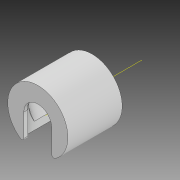
# Autodesk Inventor part: leur adapter2
Saved by Autodesk Inventor 2020 (Build 240168000, 168)
## iProperties
Created: 2020-08-02
Part Number: leur adapter2
Material: Generic
Document SubType Name: Modeling
Designer: DDeGo
Density: 1 g/cm^3
Appearance: Default
Author: DDeGo
Autodesk Inventor part; units mm, degrees
ref_plane "YZ Plane" through (0, 0, 0) normal (1, 0, 0) x (0, 1, 0)
ref_plane "XZ Plane" through (0, 0, 0) normal (0, 1, 0) x (-1, 0, 0)
ref_plane "XY Plane" through (0, 0, 0) normal (0, 0, 1) x (1, 0, 0)
sketch "Sketch1" plane through (0, 0, 0) normal (1, 0, 0) x (0, 1, 0)
  line L0 (0, 0) -> (3.6, 0) construction
  line L1 (5.6, 0) -> (5.6, -3)
  line L2 (5.6, -3) -> (3.6, -3)
  line L3 (3.6, -3) -> (3.6, 0)
  line L4 (0, 0) -> (0, -3) construction
  line L5 (0, -3) -> (3.6, -3) construction
  line L6 (3.6, 0) -> (5.6, 0)
  line L7 (4.5, 0) -> (4.5, 4.5057)
  line L8 (4.5, 6.1) -> (2.6, 6.1) construction
  line L9 (2.6, 6.1) -> (2.6, 7.1)
  line L10 (2.6, 7.1) -> (5.6, 7.1)
  line L11 (5.6, 7.1) -> (5.6, 0)
  line L12 (2.6, 6.1) -> (4.5, 4.5057)
  line L13 (4.5, 4.5057) -> (4.5, 6.1) construction
  dimension "d6" = 3.6
  dimension "d7" = 2
  dimension "d30" = 3
  dimension "d31" = 6.1
  dimension "d32" = 2.6
  dimension "d33" = 4.5
  dimension "d34" = 1
  dimension "d40" = 40
  constraints: 28 end point, 9 perpendicular, 3 vertical, 2 horizontal, 1 point on line
  measures "d6" distance between parallel lines of L4 L3
  measures "d7" distance between parallel lines of L1 L3
  measures "d30" distance of L2.end L0.end
  measures "d31" distance of L7.start L8.start
  measures "d32" distance between parallel lines of L4 L9
  measures "d33" distance between parallel lines of L4 L7
  measures "d34" distance between parallel lines of L8 L10
  measures "d40" angle of L8 L12
revolve "Revolution1" add sketch "Sketch1" angle 360 about axis through (0, 0, 0) along (0, 0, -1)
sketch "Sketch2" plane through (0, 0, 0) normal (0, 1, 0) x (-1, 0, 0)
  line L0 (-3.6, -3) -> (3.6, -3) projected
  line L1 (3.6, -3) -> (3.6, -4.7)
  line L2 (3.6, -4.7) -> (4.3, -4.2959)
  line L3 (4.3, -4.2959) -> (4.3, -3.4041)
  line L4 (4.3, -3.4041) -> (3.6, -3)
  point P0 (0, 0)
  dimension "d11" = 0.7
  dimension "d12" = 120
  dimension "d13" = 1.7
  constraints: 8 end point, 1 equal length, 1 parallel, 1 vertical
  measures "d11" distance between parallel lines of L3 L1
  measures "d12" angle of L3 L4
  measures "d13" distance of L0.end L1.end
coil "Coil1" sketch "Sketch2" operation cut axis through (0, 0, -1.5) along (0, 0, 1) pitch 7 turns 0.857143 hand right
pattern_circular "Circular Pattern1" count 2 over 360 about axis through (0, 0, -1.5) along (0, 0, -1) of "Coil1"
sketch "Sketch4" plane through (0, 0, 0) normal (0, 1, 0) x (-1, 0, 0)
  line L0 (3.25, 0) -> (-3.25, 0)
  line L1 (-3.25, 0) -> (-3.25, 8.1)
  line L2 (-3.25, 8.1) -> (3.25, 8.1)
  line L3 (3.25, 8.1) -> (3.25, 0)
  line L4 (-2.6, 7.1) -> (2.6, 7.1) projected
  line L5 (0, 8.1) -> (0, 7.1) construction
  point P0 (0, 0)
  point P1 (-2.6, 6.1)
  point P2 (2.6, 6.1)
  point P3 (-1.7059, 0)
  dimension "d35" = 6.5
  dimension "d36" = 1
  constraints: 10 end point, 2 midpoint, 2 parallel, 1 horizontal, 1 perpendicular, 1 point on line, 1 vertical
  measures "d35" distance of L1.end L2.end
  measures "d36" distance between parallel lines of L2 L4
extrude "Extrusion2" cut sketch "Sketch4" against normal blind 10
ref_plane "Work Plane1" through (2.6, 0, 6.1) normal (0, 0, 1) x (1, 0, 0)
sketch "Sketch5" plane through (2.6, 0, 6.1) normal (0, 0, 1) x (1, 0, 0)
  circle A0 centre (-2.6, 0) radius 3.25
  point P0 (-2.6, 0)
  point P1 (0.65, 0)
  constraints: 1 coincident, 1 horizontal alignment, 2 other
extrude "Extrusion3" cut sketch "Sketch5" against normal blind 2
sketch "Sketch6" plane through (0, 0, 0) normal (0, -1, 0) x (1, 0, 0)
  line L0 (-3.25, 6.1) -> (-2.6, 6.1) projected
  line L1 (-2.6, 7.1) -> (-2.6, 6.1) projected
  line L2 (-3.25, 7.1) -> (-2.6, 7.1) projected
  line L3 (-3.25, 6.1) -> (-3.25, 7.1) projected
  line L4 (2.6, 6.1) -> (3.25, 6.1) projected
  line L5 (3.25, 7.1) -> (3.25, 6.1) projected
  line L6 (2.6, 7.1) -> (3.25, 7.1) projected
  line L7 (2.6, 6.1) -> (2.6, 7.1) projected
  point P0 (0, 0)
extrude "Extrusion4" add sketch "Sketch6" along normal up to surface round surface about axis through (0, 0, 2.05) along (0, 0, -1) radius 5.6 far side no
fillet "Fillet1" radius 0.4 5 edges at (2.6, -4.9598, 6.6) (-2.6, -4.9598, 6.6) (2.6, -2.4799, 6.1) (-2.6, -2.4799, 6.1) (0, 2.6, 6.1)
body "Solid1"
